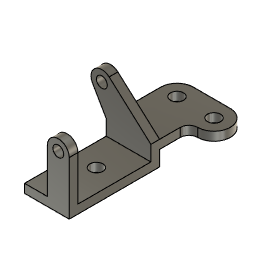
NCV-19 v2 (Autodesk Fusion 360 design; units mm, degrees)
Autodesk Fusion 360 part; units mm, degrees
sketch "Sketch1" plane through (0, 0, 0) normal (0, 0, 1) x (1, 0, 0)
  line L0 (0, 0) -> (82, 0)
  line L1 (82, 0) -> (82, -150)
  line L2 (82, -150) -> (0, -150)
  line L3 (0, -150) -> (0, 0)
  line L4 (0, 0) -> (82, 0)
  line L5 (82, 0) -> (82, 100) construction
  line L6 (82, 100) -> (0, 100) construction
  line L7 (0, 100) -> (0, 0)
  line L8 (0, 16) -> (82, 16)
  line L9 (82, 0) -> (82, 16)
  circle A0 centre (30, 100) radius 12
  circle A1 centre (98, 100) radius 12
  line L10 (30, 130) -> (98, 130)
  line L11 (82, 16) -> (82, 54)
  arc A2 (98, 70) -> (82, 54) centre (98, 54) ccw
  arc A3 (98, 70) -> (98, 130) centre (98, 100) ccw
  arc A4 (30, 130) -> (0, 100) centre (30, 100) ccw
  circle A5 centre (41, -59) radius 12
  dimension "d1" = 150
  dimension "d2" = 82
  dimension "d3" = 82
  dimension "d4" = 100
  dimension "d5" = 16
  dimension "d6" = 24
  dimension "d7" = 24
  dimension "d8" = 30
  dimension "d9" = 98
  dimension "d10" = 60
  dimension "d11" = 60
  dimension "d12" = 32
  dimension "d23" = 24
  dimension "d24" = 41
  dimension "d25" = 59
  constraint horizontal L0
  constraint vertical L1
  constraint horizontal L2
  constraint vertical L3
  constraint coincident L0.start L3.end
  constraint horizontal L4
  constraint vertical L5
  constraint horizontal L6
  constraint vertical L7
  constraint coincident L7 L8.start
  constraint coincident L5 L8.end
  constraint horizontal L8
  constraint coincident L6 A0.centre
  constraint coincident L6 A1.centre
  constraint concentric A0 A4
  constraint concentric A1 A3
  constraint horizontal L10
  constraint tangent L10 A4
  constraint vertical L11
  constraint tangent L11 A2
  constraint tangent A2 A3
  constraint coincident L5 L11.end
  measures "d1" distance of L0.start L2.end
  measures "d2" distance of L0.start L0.end
  measures "d3" distance of L0.start L0.end
  measures "d4" distance of L0.start L6.end
  measures "d5" distance of L0.start L8.start
  measures "d6" diameter of A0
  measures "d7" diameter of A1
  measures "d8" horizontal distance of L0.start A0.centre
  measures "d9" horizontal distance of L0.start A1.centre
  measures "d10" diameter of A4
  measures "d11" diameter of A3
  measures "d12" diameter of A2
  measures "d23" diameter of A5
  measures "d24" horizontal distance of L0.start A5.centre
  measures "d25" vertical distance of L0.start A5.centre
sketch "Sketch2" plane through (0, 0, 0) normal (0, 1, 0) x (1, 0, 0)
  line L0 (42, -82) -> (82, -82) construction
  line L1 (82, -82) -> (82, 0)
  line L2 (82, 0) -> (42, 0)
  line L3 (42, 0) -> (42, -82)
  circle A0 centre (-8, -82) radius 10
  circle A1 centre (62, -82) radius 10
  line L4 (0, -28) -> (82, -28)
  line L5 (0, -28) -> (-25.3346, -72.0245)
  line L6 (82, -28) -> (5.3693, -96.8748)
  arc A2 (-25.3346, -72.0245) -> (5.3693, -96.8748) centre (-8, -82) ccw
  arc A3 (42, -82) -> (82, -82) centre (62, -82) ccw
  dimension "d26" = 42
  dimension "d27" = 82
  dimension "d28" = 82
  dimension "d29" = 82
  dimension "d30" = 20
  dimension "d31" = 62
  dimension "d32" = 20
  dimension "d33" = 40
  dimension "d34" = 82
  dimension "d35" = 82
  dimension "d36" = 28
  dimension "d38" = 82
  dimension "d39" = 8
  constraint horizontal L0
  constraint vertical L1
  constraint horizontal L2
  constraint vertical L3
  constraint coincident L0 A1.centre
  constraint tangent L1 A3
  constraint concentric A0 A2
  constraint horizontal L4
  constraint tangent L5 A2
  constraint tangent L6 A2
  measures "d26" horizontal distance of L2.end origin
  measures "d27" horizontal distance of L1.end origin
  measures "d28" vertical distance of L0.start origin
  measures "d29" distance of L0.start L2.end
  measures "d30" diameter of A1
  measures "d31" horizontal distance of origin A1.centre
  measures "d32" diameter of A0
  measures "d33" diameter of A2
  measures "d34" horizontal distance of origin L4.end
  measures "d35" distance of L4.start L4.end
  measures "d36" distance of origin L4.start
  measures "d38" vertical distance of A0.centre origin
  measures "d39" horizontal distance of A0.centre origin
extrude "Extrude1" add sketch "Sketch1" against normal blind 16 contours L0 L1 L2 L3 L4
extrude "Extrude2" add sketch "Sketch1" along normal blind 28 and the other way up to surface (16 mm away) contours L0 L4 L7 L8 L9
extrude "Extrude3" add sketch "Sketch1" along normal blind 16 from surface at 12 contours L7 L8 L10 L11 A2 A3 A4
extrude "Extrude5" add sketch "Sketch2" along normal blind 16 from surface at -150 contours L1 L3 L6 A3 | L1 L2 L3 L4 | L3 L4 L6
extrude "Extrude6" add sketch "Sketch2" along normal blind 16 contours L3 L4 L6 | L3 L4 L5 L6 A2
equation "d3 = d2"
equation "d4 = 84 mm + 16 mm"
equation "d9 = d8 + 68 mm"
equation "d25 = 150 mm - 16 mm - 16 mm - 59 mm"
equation "d31 = 42 mm + ( 82 - 42 ) / 2 * 1 mm"
equation "d45 = 28 mm - 16 mm"
